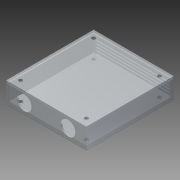
# Autodesk Inventor part: Enclosure
Saved by Autodesk Inventor 2015 (Build 190159000, 159)
## iProperties
Created: 2014-08-04
Part Number: Enclosure
Material: Glass
Document SubType Name: Modeling
Designer: Patrick Camilleri
Density: 2.18 g/cm^3
Appearance: Clear
Mass: 1670.93 g
Surface Area: 3005.46 cm^2
Volume: 766.481 cm^3
Author: Patrick Camilleri
Autodesk Inventor part; units mm, degrees
ref_plane "YZ Plane" through (0, 0, 0) normal (1, 0, 0) x (0, 1, 0)
ref_plane "XZ Plane" through (0, 0, 0) normal (0, 1, 0) x (-1, 0, 0)
ref_plane "XY Plane" through (0, 0, 0) normal (0, 0, 1) x (1, 0, 0)
sketch "Sketch2" plane through (0, 0, 0) normal (0, 0, 1) x (1, 0, 0)
  line L0 (0, 0) -> (220, 0)
  line L1 (220, 0) -> (220, -240)
  line L2 (220, -240) -> (0, -240)
  line L3 (0, -240) -> (0, 0)
  dimension "d0" = 240
  dimension "d1" = 220
  constraints: 8 end point, 2 parallel, 1 horizontal, 1 perpendicular
  measures "d0" distance of L2.end L0.start
  measures "d1" distance of L0.start L0.end
extrude "Extrusion1" add sketch "Sketch2" along normal blind 50
sketch "Sketch3" plane through (0, 0, 50) normal (0, 0, 1) x (1, 0, 0)
  line L0 (4, -4) -> (216, -4)
  line L1 (216, -4) -> (216, -236)
  line L2 (216, -236) -> (4, -236)
  line L3 (4, -236) -> (4, -4)
  line L4 (0, 0) -> (0, -240) projected
  line L5 (220, -240) -> (220, 0) projected
  line L6 (0, -240) -> (220, -240) projected
  line L7 (220, 0) -> (0, 0) projected
  dimension "d4" = 4
  dimension "d5" = 4
  dimension "d6" = 4
  dimension "d7" = 4
  constraints: 8 end point, 2 parallel, 1 horizontal, 1 perpendicular
  measures "d4" distance between parallel lines of L3 L4
  measures "d5" distance between parallel lines of L5 L1
  measures "d6" distance between parallel lines of L2 L6
  measures "d7" distance between parallel lines of L7 L0
extrude "Extrusion2" cut sketch "Sketch3" against normal blind 44 contours L0 L1 L2 L3
ref_plane "Work Plane1" through (220, -240, 50) normal (0, 0, 1) x (1, 0, 0)
sketch "Sketch4" plane through (220, -240, 50) normal (0, 0, 1) x (1, 0, 0)
  line L0 (-220, 0) -> (0, 0) projected
  line L1 (-220, 240) -> (-220, 0) projected
  line L2 (0, 0) -> (0, 240) projected
  line L3 (0, 240) -> (-220, 240) projected
extrude "Extrusion3" add sketch "Sketch4" along normal blind 6 separate body
ref_plane "Work Plane2" through (220, 0, 56) normal (0, 0, 1) x (1, 0, 0)
sketch "Sketch6" plane through (220, 0, 56) normal (0, 0, 1) x (1, 0, 0)
  line L0 (-220, 0) -> (-220, -240) projected
  line L1 (0, 0) -> (-220, 0) projected
  point P0 (-200, -20)
  point P1 (-20, -20)
  point P2 (-200, -220)
  point P3 (-20, -220)
  dimension "d12" = 20
  dimension "d13" = 20
  dimension "d16" = 180
  dimension "d19" = 200
  constraints: 1 horizontal, 1 vertical, 3 other
  measures "d12" distance from line of L0 point (-200, -20)
  measures "d13" distance from line of L1 point (-200, -20)
  measures "d16" distance of point (-200, -20) point (-20, -20)
  measures "d19" distance of point (-200, -20) point (-200, -220)
hole "Hole1" at (20, -20, 56) at (200, -20, 56) at (20, -220, 56) at (200, -220, 56) direction (0, 0, -1) diameter 10 end through all bodies 2
ref_plane "Work Plane3" through (0, 0, 0) normal (0, 0, -1) x (-1, 0, 0)
sketch "Sketch7" plane through (0, 0, 0) normal (0, 0, -1) x (-1, 0, 0)
  circle A0 centre (-200, -220) radius 5 projected
  circle A1 centre (-20, -220) radius 5 projected
  circle A2 centre (-20, -20) radius 5 projected
  circle A3 centre (-200, -20) radius 5 projected
  point P0 (0, 0)
extrude "Extrusion4" cut sketch "Sketch7" against normal blind 6 bodies 1
ref_plane "Work Plane4" through (220, -240, 0) normal (0, -1, 0) x (1, 0, 0)
sketch "Sketch8" plane through (220, -240, 0) normal (0, -1, 0) x (1, 0, 0)
  circle A0 centre (-170, 27.5) radius 20
  circle A1 centre (-50, 27.5) radius 20
  line L0 (-220, 0) -> (-220, 50) projected
  line L1 (0, 0) -> (0, 50) projected
  line L2 (0, 0) -> (-220, 0) projected
  dimension "d31" = 40
  dimension "d32" = 40
  dimension "d33" = 50
  dimension "d34" = 50
  dimension "d35" = 27.5
  constraints: 2 centre point, 1 horizontal alignment
  measures "d31" diameter of A0
  measures "d32" diameter of A1
  measures "d33" distance from line of A0.centre L0
  measures "d34" distance from line of A1.centre L1
  measures "d35" distance from line of L2 A0.centre
extrude "Extrusion5" cut sketch "Sketch8" against normal blind 6 bodies 1
ref_plane "Work Plane5" through (220, 0, 0) normal (0, 1, 0) x (1, 0, 0)
sketch "Sketch9" plane through (220, 0, 0) normal (0, 1, 0) x (1, 0, 0)
  line L0 (-210, -40) -> (-10, -40)
  line L1 (-10, -40) -> (-10, -37)
  line L2 (-10, -37) -> (-210, -37)
  line L3 (-210, -37) -> (-210, -40)
  line L4 (-210, -32) -> (-10, -32)
  line L5 (-10, -32) -> (-10, -29)
  line L6 (-10, -29) -> (-210, -29)
  line L7 (-210, -29) -> (-210, -32)
  line L8 (-210, -24) -> (-10, -24)
  line L9 (-10, -24) -> (-10, -21)
  line L10 (-10, -21) -> (-210, -21)
  line L11 (-210, -21) -> (-210, -24)
  line L12 (-210, -16) -> (-10, -16)
  line L13 (-10, -16) -> (-10, -13)
  line L14 (-10, -13) -> (-210, -13)
  line L15 (-210, -13) -> (-210, -16)
  line L16 (0, -50) -> (-220, -50) projected
  line L17 (0, 0) -> (0, -50) projected
  line L18 (-220, 0) -> (-220, -50) projected
  line L19 (-10, -8) -> (-210, -8)
  line L20 (-210, -8) -> (-210, -5)
  line L21 (-210, -5) -> (-10, -5)
  line L22 (-10, -5) -> (-10, -8)
  point P0 (-10, -38.5)
  point P1 (-10, -30.5)
  point P2 (-10, -22.5)
  point P3 (-10, -14.5)
  point P4 (-10, -6.5)
  dimension "d38" = 3
  dimension "d39" = 3
  dimension "d40" = 3
  dimension "d41" = 3
  dimension "d42" = 5
  dimension "d43" = 5
  dimension "d44" = 5
  dimension "d45" = 10
  dimension "d46" = 10
  dimension "d48" = 200
  dimension "d50" = 3
  dimension "d51" = 5
  constraints: 40 end point, 10 parallel, 6 point on line, 5 horizontal, 5 midpoint, 5 perpendicular, 3 vertical alignment
  measures "d38" distance of L0.end L1.end
  measures "d39" distance of L4.end L5.end
  measures "d40" distance of L8.end L9.end
  measures "d41" distance of L12.end L13.end
  measures "d42" distance between parallel lines of L4 L2
  measures "d43" distance between parallel lines of L8 L6
  measures "d44" distance between parallel lines of L12 L10
  measures "d45" distance between parallel lines of L16 L0
  measures "d46" distance between parallel lines of L17 L1
  measures "d48" distance of L0.start L0.end
  measures "d50" distance of L21.end L19.start
  measures "d51" distance between parallel lines of L19 L14
extrude "Extrusion6" cut sketch "Sketch9" against normal blind 6 bodies 1
equation "\"d5\" = d4"
equation "\"d6\" = d4"
equation "\"d7\" = d4"
equation "\"d13\" = d12"
equation "\"d32\" = d31"
equation "\"d34\" = d33"
equation "\"d39\" = d38"
equation "\"d40\" = d38"
equation "\"d41\" = d38"
equation "\"d50\" = d38"
body "Solid1"
body "Solid2"
